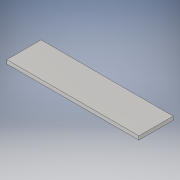
# Autodesk Inventor part: blech_optic
Saved by Autodesk Inventor 2017 (Build 210142000, 142)
## iProperties
Part Number: blech_optic
Material: Generisch
Document SubType Name: Modeling
Designer: Philomena-Theresa
Density: 1 g/cm^3
Appearance: Vorgabe
Author: Philomena-Theresa
Autodesk Inventor part; units mm, degrees
ref_plane "YZ Plane" through (0, 0, 0) normal (1, 0, 0) x (0, 1, 0)
ref_plane "XZ Plane" through (0, 0, 0) normal (0, 1, 0) x (-1, 0, 0)
ref_plane "XY Plane" through (0, 0, 0) normal (0, 0, 1) x (1, 0, 0)
sketch "Skizze1" plane through (0, 0, 0) normal (0, 0, 1) x (1, 0, 0)
  line L0 (-38.5, 10) -> (38.5, 10)
  line L1 (38.5, 10) -> (38.5, -10)
  line L2 (38.5, -10) -> (-38.5, -10)
  line L3 (-38.5, -10) -> (-38.5, 10)
  line L4 (-38.5, 10) -> (38.5, -10) construction
  point P0 (0, 0)
  point P1 (0, 0)
  dimension "d0" = 77
  dimension "d1" = 20
  constraints: 10 end point, 2 parallel, 1 coincident, 1 horizontal, 1 midpoint, 1 perpendicular
  measures "d0" distance of L1.end L2.end
  measures "d1" distance of L0.end L1.end
extrude "Extrusion1" add sketch "Skizze1" along normal blind 2.17
